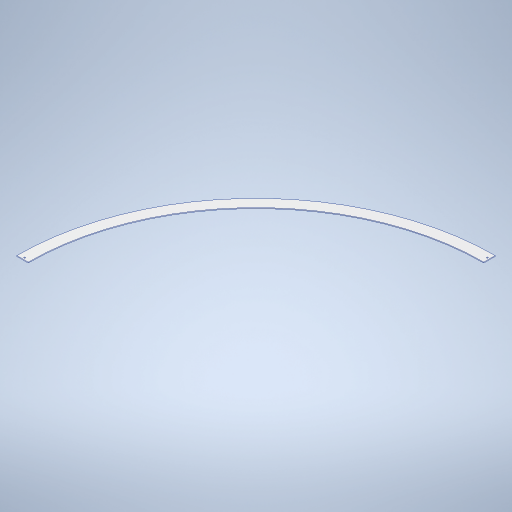
# Autodesk Inventor part: Arco menor
Saved by Autodesk Inventor 2024 (Build 280153000, 153)
## iProperties
Created: 2024-05-02
Part Number: Arco menor
Material: Alumínio 6061
Document SubType Name: Modeling
Designer: mathe
Density: 2.7 g/cm^3
Appearance: Alumínio - Plano
Author: mathe
Autodesk Inventor part; units mm, degrees
ref_plane "YZ Plane" through (0, 0, 0) normal (1, 0, 0) x (0, 1, 0)
ref_plane "XZ Plane" through (0, 0, 0) normal (0, 1, 0) x (-1, 0, 0)
ref_plane "XY Plane" through (0, 0, 0) normal (0, 0, 1) x (1, 0, 0)
sketch "Esboço1" plane through (0, 0, 0) normal (0, 1, 0) x (-1, 0, 0)
  arc A0 (0, -805) -> (805, 0) centre (0, 0) ccw
  arc A1 (0, -845) -> (845, 0) centre (0, 0) ccw
  line L0 (805, 0) -> (845, 0)
  line L1 (0, -805) -> (0, -845)
  circle A2 centre (7.5, -815) radius 2.5
  circle A3 centre (7.5, -835) radius 2.5
  circle A4 centre (835, -7.5) radius 2.5
  circle A5 centre (815, -7.5) radius 2.5
  circle A6 centre (835, -7.5) radius 2.5
  circle A7 centre (815, -7.5) radius 2.5
  dimension "d0" = 805
  dimension "d1" = 845
  dimension "d2" = 5
  dimension "d3" = 5
  dimension "d4" = 20
  dimension "d6" = 7.5
  dimension "d7" = 5
  dimension "d8" = 5
  dimension "d9" = 7.5
  dimension "d10" = 10
  dimension "d11" = 20
  dimension "d13" = 7.5
  dimension "d14" = 7.5
  dimension "d15" = 10
  constraints: 8 centre point, 4 coincident, 4 end point, 4 point on circle, 2 concentric, 1 horizontal, 1 perpendicular
  measures "d0" radius of A0
  measures "d1" radius of A1
  measures "d2" diameter of A2
  measures "d3" diameter of A3
  measures "d4" distance of A3.centre A2.centre
  measures "d6" distance from line of L1 A2.centre
  measures "d7" diameter of A4
  measures "d8" diameter of A5
  measures "d9" distance from line of L0 A5.centre
  measures "d10" horizontal distance of L0.end A4.centre
  measures "d11" distance of A5.centre A4.centre
  measures "d13" distance from line of L0 A4.centre
  measures "d14" distance from line of L1 A3.centre
  measures "d15" vertical distance of L1.end A3.centre
extrude "Extrusão1" add sketch "Esboço1" along normal blind 3 contours A0 L0 A1 L1 | A2 | A3 | A4 | A5
sketch "Esboço4" plane through (0, 3, 0) normal (0, 1, 0) x (1, 0, 0)
  circle A0 centre (-825, 7.5) radius 2.5
  line L0 (-845, 0) -> (-805, 0) projected
  circle A1 centre (-7.5, 825) radius 2.5
  line L1 (0, 805) -> (0, 845) projected
  point P0 (0, 0)
  dimension "d19" = 5
  dimension "d22" = 7.5
  dimension "d25" = 5
  dimension "d26" = 7.5
  dimension "d44" = 20
  dimension "d45" = 20
  constraints: 2 centre point
  measures "d19" diameter of A0
  measures "d22" distance from line of L0 A0.centre
  measures "d25" diameter of A1
  measures "d26" distance from line of L1 A1.centre
  measures "d44" horizontal distance of L0.end A0.centre
  measures "d45" vertical distance of A1.centre L1.end
hole "Furo1" at (-825, 3, -7.5) at (-7.5, 3, -825) direction (0, -1, 0) diameter 5 end through all
